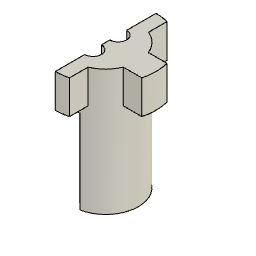
4pole_dipole (Autodesk Fusion 360 design; units mm, degrees)
Autodesk Fusion 360 part; units mm, degrees
sketch "Sketch1" plane through (0, 0, 0) normal (0, 0, 1) x (1, 0, 0)
  circle A0 centre (0, 0) radius 3.9
  circle A1 centre (0, 1.5) radius 1
  line L0 (-3.5, 0) -> (3.5, 0) construction
  circle A2 centre (0, -1.5) radius 1
  line L1 (0, 3.9) -> (0, -3.9) construction
  dimension "d1" = 7.8
  dimension "d2" = 2
  constraint coincident A0.centre origin
  constraint horizontal L0
  constraint symmetric A1 L0 A2
  constraint vertical L1
  constraint coincident A0 L1.end
  constraint coincident A0 L1.start
  measures "d1" diameter of A0
  measures "d2" diameter of A1
extrude "Extrude1" add sketch "Sketch1" along normal blind 15
sketch "Sketch2" plane through (0, 0, 0) normal (0, 0, -1) x (1, 0, 0)
  circle A0 centre (0, 1.5) radius 1
  circle A1 centre (0, -1.5) radius 1
  circle A2 centre (0, 0) radius 3.9
  circle A3 centre (0, 1.5) radius 1.3
  circle A4 centre (0, -1.5) radius 1.3
  circle A5 centre (0, 1) radius 0.15
  line L0 (1.75, 0) -> (22.5, 0)
  circle A6 centre (0, -1) radius 0.15
  dimension "d7" = 0.3
  dimension "d8" = 2
  constraint concentric A0 A3
  constraint concentric A1 A4
  constraint symmetric A5 L0 A6
  measures "d7" diameter of A5
  measures "d8" distance of A5.centre A6.centre
extrude "Extrude2" add sketch "Sketch2" against normal blind 2 contours A0 | A1 | A3 | A4
sketch "Sketch3" plane through (0, 0, 15) normal (0, 0, 1) x (-1, 0, 0)
  circle A0 centre (0, 1.5) radius 1
  circle A1 centre (0, -1.5) radius 1
  circle A2 centre (0, 0) radius 3.9
  line L0 (0, 0) -> (0, -5)
  line L1 (0, -5) -> (5, -5)
  line L2 (5, -5) -> (5, 5)
  line L3 (5, 5) -> (0, 5)
  line L4 (0, 5) -> (0, 0)
  constraint coincident A2.centre L0.start
  constraint vertical L0
  constraint perpendicular L0 L1
  constraint perpendicular L1 L2
  constraint perpendicular L2 L3
  constraint perpendicular L3 L4
extrude "Extrude3" cut sketch "Sketch3" against normal blind 26 contours A0 L4 | A0 A1 A2 L0 L4 | A1 L0 picked at (0.2519, 1.7183) picked at (1.8608, 0) picked at (0.2519, -1.2817)
sketch "Sketch4" plane through (0, 0, 15) normal (0, 0, 1) x (-1, 0, 0)
  line L0 (0, -0.5) -> (0, 0.5)
  arc A0 (0, 2.5) -> (0, 0.5) centre (0, 1.5) ccw
  line L1 (0, 2.5) -> (0, 3.9)
  arc A1 (0, 3.9) -> (0, -3.9) centre (0, 0) ccw
  line L2 (0, -3.9) -> (0, -2.5)
  arc A2 (0, -0.5) -> (0, -2.5) centre (0, -1.5) ccw
  line L3 (0.5904, -3.3483) -> (0.6776, -3.8427)
  line L4 (0, 0.3395) -> (-0.0009, 0.3446)
  arc A3 (0, -3.9) -> (0.6776, -3.8427) centre (0.0085, 0.0338) ccw
  arc A4 (0, 3.3) -> (-0.0002, 3.3) centre (0, 0) ccw
  line L5 (-0.6694, 3.2314) -> (-0.7736, 3.8225)
  line L6 (0.5904, -3.3483) -> (0.5383, -3.0529)
  line L7 (-0.6694, 3.2314) -> (-0.6347, 3.0343)
  arc A5 (0, 3.1) -> (-0.6347, 3.0343) centre (0, 0) ccw
  arc A6 (0, -3.1) -> (0.5383, -3.0529) centre (0, 0) ccw
  line L8 (0, 3.1) -> (0, 3.9)
  dimension "d28" = 6.2
  constraint coincident A1 L5.end
  constraint concentric A4 A5
  constraint parallel L3 L6
  constraint parallel L5 L7
  constraint coincident L1 A5.start
  constraint coincident L0 L4.start
  constraint coincident L2 A6.start
  constraint concentric A5 A6
  constraint coincident L1.end A1.start
  measures "d28" diameter of A5
extrude "Extrude4" add sketch "Sketch4" against normal blind 10 from surface at -5 contours L2 A4 L6 A6 | L2 L3 A3 A4 L6 | L1 A1 A4 L5 L8 | L1 A4 L7 A5 L8
extrude "Extrude5" cut sketch "Sketch4" against normal blind 10 from surface at -5 contours L1 A1 A4 L5 L8 | L1 A4 L7 A5 L8
sketch "Sketch5" plane through (0, 0, 15) normal (0, 0, 1) x (-1, 0, 0)
  line L0 (0, -0.5) -> (0, 0.5)
  arc A0 (0, 2.5) -> (0, 0.5) centre (0, 1.5) ccw
  arc A1 (0, 3.9) -> (0, -3.9) centre (0, 0) ccw
  arc A2 (0, -0.5) -> (0, -2.5) centre (0, -1.5) ccw
  line L1 (-5.2915, -1.5) -> (-3.6, -1.5)
  line L2 (-5.2915, 1.5) -> (-3.6, 1.5)
  line L3 (-5.2915, -1.5) -> (-5.8095, -1.5)
  line L4 (-5.2915, 1.5) -> (-5.8095, 1.5)
  line L5 (0, -3.9) -> (0, -6)
  line L6 (0, 3.9) -> (0, 6)
  line L7 (-1.5, 5.2915) -> (-1.5, 5.8095)
  arc A3 (-1.5, -5.8095) -> (0, -6) centre (0, 0) ccw
  arc A4 (0, 6) -> (-1.5, 5.8095) centre (0, 0) ccw
  arc A5 (-5.8095, 1.5) -> (-5.8095, -1.5) centre (0, 0) ccw
  line L8 (0, 2.5) -> (0, 3.9)
  line L9 (0, -3.9) -> (0, -2.5)
  arc A6 (-5.8095, 1.5) -> (-5.8095, -1.5) centre (0, 0) ccw
  arc A7 (-1.5, -5.8095) -> (0, -6) centre (0, 0) ccw
  arc A8 (0, 6) -> (-1.5, 5.8095) centre (0, 0) ccw
  line L10 (-1.5, 5.2915) -> (-1.5, 3.6)
  line L11 (-1.5, -3.6) -> (-1.5, -5.8095)
  arc A9 (-1.5, -3.6) -> (0, -3.9) centre (0, 0) ccw
  arc A10 (0, 3.9) -> (-1.5, 3.6) centre (0, 0) ccw
  arc A11 (-3.6, 1.5) -> (-3.6, -1.5) centre (0, 0) ccw
  point P0 (-0.8888, 0)
  dimension "d30" = 1.5
  dimension "d31" = 1.5
  constraint parallel L1 L2
  constraint perpendicular L2 L10
  constraint parallel L1 L3
  constraint coincident L4.end A4
  constraint parallel L2 L4
  constraint parallel L7 L10
  constraint concentric A3 A4
  constraint concentric A4 A5
  constraint concentric A4 A7
  constraint concentric A5 A10
  constraint vertical L10
  constraint coincident A1 L1.end
  constraint concentric A6 A7
  constraint coincident A1 L2.end
  constraint concentric A7 A8
  constraint coincident A1 L10.end
  constraint coincident A1 L11.start
  constraint collinear L10 L11
  constraint concentric A9 A10
  constraint concentric A10 A11
  constraint coincident A1.end L5.start
  constraint coincident A1.start L6.start
  measures "d30" distance of L1 A1.centre
  measures "d31" distance of L2 A1.centre
extrude "Extrude6" add sketch "Sketch5" against normal blind 4 contours A1 L5 A3 A7 L11 A9 | A1 L6 L7 A4 A8 L10 A10 | A1 L1 L2 L3 L4 A5 A6 A11
extrude "Extrude7" cut 1 faces at (-0.5563, 3.5901, 10) along direction (0, 0, -1) blind 0.1
